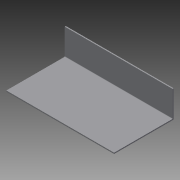
# Autodesk Inventor part: supply base
Saved by Autodesk Inventor 2015 (Build 190159000, 159)
## iProperties
Created: 2015-01-31
Part Number: supply base
Material: Generic
Document SubType Name: Modeling
Designer: Joseph
Density: 1 g/cm^3
Appearance: Default
Author: Joseph
Autodesk Inventor part; units mm, degrees
ref_plane "YZ Plane" through (0, 0, 0) normal (1, 0, 0) x (0, 1, 0)
ref_plane "XZ Plane" through (0, 0, 0) normal (0, 1, 0) x (-1, 0, 0)
ref_plane "XY Plane" through (0, 0, 0) normal (0, 0, 1) x (1, 0, 0)
sketch "Sketch2" plane through (0, 0, 0) normal (0, 0, 1) x (1, 0, 0)
  line L0 (99.5, 55) -> (-99.5, 55)
  line L1 (-99.5, 55) -> (-99.5, -55)
  line L2 (-99.5, -55) -> (99.5, -55)
  line L3 (99.5, -55) -> (99.5, 55)
  line L4 (99.5, 55) -> (-99.5, -55) construction
  line L5 (-99.5, 55) -> (99.5, -55) construction
  point P0 (0, 0)
  dimension "d4" = 199
  dimension "d5" = 110
  constraints: 12 end point, 2 midpoint, 2 parallel, 1 horizontal, 1 perpendicular
  measures "d4" distance of L2.end L1.end
  measures "d5" distance of L1.end L0.end
extrude "Extrusion2" add sketch "Sketch2" along normal blind 2
sketch "Sketch3" plane through (0, 0, 2) normal (0, 0, 1) x (1, 0, 0)
  line L0 (99.5, -55) -> (99.5, 55) projected
  line L1 (-99.5, 55) -> (99.5, 55)
  line L2 (99.5, 55) -> (99.5, 53)
  line L3 (99.5, 53) -> (-99.5, 53)
  line L4 (-99.5, 53) -> (-99.5, 55)
  point P0 (0, 0)
  dimension "d8" = 2
  constraints: 8 end point, 2 parallel, 1 horizontal, 1 perpendicular, 1 point on line
  measures "d8" distance of L1.end L2.end
extrude "Extrusion3" add sketch "Sketch3" along normal blind 48
fillet "Fillet1" radius 1 2 edges at (0, 55, 0) (0, 53, 2)
body "Solid2"
